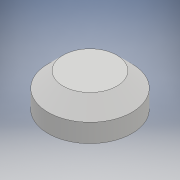
# Autodesk Inventor part: bolt_Prop
Saved by Autodesk Inventor 2018 (Build 220112000, 112)
## iProperties
Created: 2019-02-05
Part Number: bolt_Prop
Material: Generic
Document SubType Name: Modeling
Designer: JARVIS
Density: 1 g/cm^3
Appearance: Default
Author: JARVIS
Autodesk Inventor part; units mm, degrees
ref_plane "YZ Plane" through (0, 0, 0) normal (1, 0, 0) x (0, 1, 0)
ref_plane "XZ Plane" through (0, 0, 0) normal (0, 1, 0) x (-1, 0, 0)
ref_plane "XY Plane" through (0, 0, 0) normal (0, 0, 1) x (1, 0, 0)
sketch "Sketch1" plane through (0, 0, 0) normal (0, 0, 1) x (1, 0, 0)
  circle A0 centre (0, 0) radius 12.5
  dimension "d0" = 25
  constraints: 1 centre point, 1 coincident
  measures "d0" diameter of A0
extrude "Extrusion1" add sketch "Sketch1" along normal blind 10
sketch "Sketch2" plane through (0, 0, 0) normal (0, 0, -1) x (-1, 0, 0)
  circle A0 centre (0, 0) radius 12
  dimension "d3" = 24
  constraints: 1 centre point, 1 coincident
  measures "d3" diameter of A0
extrude "Extrusion2" cut sketch "Sketch2" against normal blind 3
sketch "Sketch4" plane through (0, 0, 3) normal (0, 0, -1) x (-1, 0, 0)
  line L0 (0, 7.7942) -> (6.75, 3.8971)
  line L1 (6.75, 3.8971) -> (6.75, -3.8971)
  line L2 (6.75, -3.8971) -> (0, -7.7942)
  line L3 (0, -7.7942) -> (-6.75, -3.8971)
  line L4 (-6.75, -3.8971) -> (-6.75, 3.8971)
  line L5 (-6.75, 3.8971) -> (0, 7.7942)
  point P0 (0, 0)
  point P1 (0, 0)
  point P2 (-6.75, 0)
  dimension "d6" = 13.5
  constraints: 12 end point, 1 coincident, 1 horizontal alignment, 1 midpoint, 13 other
  measures "d6" distance between parallel lines of L4 L1
extrude "Extrusion3" cut sketch "Sketch4" against normal blind 6
sketch "Sketch5" plane through (0, 0, 3) normal (0, 0, -1) x (-1, 0, 0)
  line L0 (-6.75, -3.8971) -> (-6.75, 3.8971) projected
  arc A0 (-6.75, -0.7) -> (-6.75, 0.7) centre (-6.75, 0) ccw
  point P0 (0, 0)
  dimension "d10" = 0.7
  constraints: 2 point on circle, 2 point on line, 1 centre point, 1 midpoint
  measures "d10" radius of A0
extrude "Extrusion4" add sketch "Sketch5" against normal blind 2
fillet "Fillet2" radius 0.7 2 edges at (6.05, 0, 3) (6.05, 0, 5)
sketch "Sketch6" plane through (0, 0, 3) normal (0, 0, -1) x (-1, 0, 0)
  line L0 (-6.75, 0) -> (-6.75, 3.8971) projected
  line L1 (-6.75, 0) -> (-6.75, -3.8971) projected
  line L2 (-8.35, 2.5) -> (-7.35, 2.5)
  line L3 (-7.35, 2.5) -> (-7.35, -2.5)
  line L4 (-7.35, -2.5) -> (-8.35, -2.5)
  line L5 (-8.35, -2.5) -> (-8.35, 2.5)
  point P0 (0, 0)
  point P1 (-7.35, 0)
  dimension "d14" = 1
  dimension "d15" = 0.6
  dimension "d16" = 5
  constraints: 8 end point, 2 parallel, 1 horizontal, 1 horizontal alignment, 1 midpoint, 1 perpendicular
  measures "d14" distance of L2.start L2.end
  measures "d15" distance between parallel lines of L3 L0
  measures "d16" distance of L4.end L2.start
extrude "Extrusion5" cut sketch "Sketch6" against normal blind 5
chamfer "Chamfer1" distance 4.5 angle 45 1 edges at (-12.5, 0, 10)
pattern_circular "Circular Pattern2" count 6 over 360 about axis through (0, 0, 0) along (0, 0, 1) of "Extrusion5", "Extrusion4", "Fillet2"
body "Solid1"
